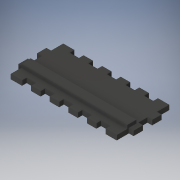
# Autodesk Inventor part: front
Saved by Autodesk Inventor 2019 (Build 230136000, 136)
## iProperties
Created: 2018-06-06
Part Number: front
Material: PBT Plastic Black
Document SubType Name: Modeling
Designer: stra92745
Density: 1.31 g/cm^3
Appearance: Smooth - White
Author: stra92745
Autodesk Inventor part; units mm, degrees
ref_plane "YZ Plane" through (0, 0, 0) normal (1, 0, 0) x (0, 1, 0)
ref_plane "XZ Plane" through (0, 0, 0) normal (0, 1, 0) x (-1, 0, 0)
ref_plane "XY Plane" through (0, 0, 0) normal (0, 0, 1) x (1, 0, 0)
sketch "Sketch1" plane through (0, 0, 0) normal (0, 1, 0) x (-1, 0, 0)
  line L0 (0, 0) -> (-99, 0)
  line L1 (-99, 0) -> (-99, -45)
  line L2 (-99, -45) -> (0, -45)
  line L3 (0, -45) -> (0, 0)
  dimension "d0" = 99
  dimension "d1" = 45
  constraints: 8 end point, 2 parallel, 1 horizontal, 1 perpendicular
  measures "d0" distance of L2.end L1.end
  measures "d1" distance of L1.end L0.end
extrude "Extrusion1" add sketch "Sketch1" along normal blind 4
sketch "Sketch2" plane through (0, 4, 0) normal (0, 1, 0) x (1, 0, 0)
  line L0 (99, 45) -> (0, 45) construction
  line L1 (99, 0) -> (99, 45) construction
  line L2 (0, 0) -> (99, 0) construction
  line L3 (0, 45) -> (0, 0) construction
  line L4 (4, 41) -> (95, 41) construction
  line L5 (95, 41) -> (95, 4) construction
  line L6 (95, 4) -> (4, 4) construction
  line L7 (4, 4) -> (4, 41) construction
  line L8 (4, 34.5) -> (0, 34.5)
  line L9 (0, 34.5) -> (0, 45)
  line L10 (0, 45) -> (4, 45)
  line L11 (4, 45) -> (4, 34.5)
  line L12 (0, 22.5) -> (99, 22.5) construction
  line L13 (49.5, 0) -> (49.5, 45) construction
  line L14 (0, 26.5) -> (4, 26.5)
  line L15 (0, 26.5) -> (0, 22.5)
  line L16 (4, 26.5) -> (4, 22.5)
  line L17 (13.5, 45) -> (13.5, 41)
  line L18 (13.5, 41) -> (21.5, 41)
  line L19 (21.5, 41) -> (21.5, 45)
  line L20 (21.5, 45) -> (13.5, 45)
  line L21 (29.5, 45) -> (29.5, 41)
  line L22 (29.5, 41) -> (37.5, 41)
  line L23 (37.5, 45) -> (37.5, 41)
  line L24 (37.5, 45) -> (29.5, 45)
  line L25 (45.5, 41) -> (45.5, 45)
  line L26 (45.5, 41) -> (49.5, 41)
  line L27 (49.5, 45) -> (45.5, 45)
  line L28 (4, 10.5) -> (0, 10.5)
  line L29 (0, 10.5) -> (0, 0)
  line L30 (0, 0) -> (4, 0)
  line L31 (4, 0) -> (4, 10.5)
  line L32 (0, 18.5) -> (4, 18.5)
  line L33 (0, 18.5) -> (0, 22.5)
  line L34 (4, 18.5) -> (4, 22.5)
  line L35 (13.5, 0) -> (13.5, 4)
  line L36 (13.5, 4) -> (21.5, 4)
  line L37 (21.5, 4) -> (21.5, 0)
  line L38 (21.5, 0) -> (13.5, 0)
  line L39 (29.5, 0) -> (29.5, 4)
  line L40 (29.5, 4) -> (37.5, 4)
  line L41 (37.5, 0) -> (37.5, 4)
  line L42 (37.5, 0) -> (29.5, 0)
  line L43 (45.5, 4) -> (45.5, 0)
  line L44 (45.5, 4) -> (49.5, 4)
  line L45 (49.5, 0) -> (45.5, 0)
  line L46 (99, 45) -> (99, 0) construction
  line L47 (95, 4) -> (95, 41) construction
  line L48 (95, 34.5) -> (99, 34.5)
  line L49 (99, 34.5) -> (99, 45)
  line L50 (99, 45) -> (95, 45)
  line L51 (95, 45) -> (95, 34.5)
  line L52 (99, 26.5) -> (95, 26.5)
  line L53 (99, 26.5) -> (99, 22.5)
  line L54 (95, 26.5) -> (95, 22.5)
  line L55 (85.5, 45) -> (85.5, 41)
  line L56 (85.5, 41) -> (77.5, 41)
  line L57 (77.5, 41) -> (77.5, 45)
  line L58 (77.5, 45) -> (85.5, 45)
  line L59 (69.5, 45) -> (69.5, 41)
  line L60 (69.5, 41) -> (61.5, 41)
  line L61 (61.5, 45) -> (61.5, 41)
  line L62 (61.5, 45) -> (69.5, 45)
  line L63 (53.5, 41) -> (53.5, 45)
  line L64 (53.5, 41) -> (49.5, 41)
  line L65 (49.5, 45) -> (53.5, 45)
  line L66 (99, 0) -> (95, 0)
  line L67 (69.5, 0) -> (69.5, 4)
  line L68 (69.5, 4) -> (61.5, 4)
  line L69 (61.5, 0) -> (69.5, 0)
  line L70 (61.5, 0) -> (61.5, 4)
  line L71 (53.5, 4) -> (53.5, 0)
  line L72 (53.5, 4) -> (49.5, 4)
  line L73 (49.5, 0) -> (53.5, 0)
  line L74 (95, 0) -> (95, 10.5)
  line L75 (95, 10.5) -> (99, 10.5)
  line L76 (99, 10.5) -> (99, 0)
  line L77 (85.5, 0) -> (85.5, 4)
  line L78 (99, 18.5) -> (95, 18.5)
  line L79 (77.5, 0) -> (85.5, 0)
  line L80 (77.5, 4) -> (77.5, 0)
  line L81 (85.5, 4) -> (77.5, 4)
  line L82 (95, 18.5) -> (95, 22.5)
  line L83 (99, 18.5) -> (99, 22.5)
  dimension "d8" = 4
  dimension "d11" = 8
  dimension "d12" = 4
  dimension "d14" = 8
  dimension "d15" = 8
  dimension "d16" = 8
  dimension "d17" = 4
  dimension "d18" = 8
  constraints: 160 end point, 49 symmetric about line, 18 point on line, 8 midpoint, 5 perpendicular, 3 collinear, 2 horizontal, 2 vertical, 1 parallel, 11 other
  measures "d11" distance between parallel lines of L14 L8
  measures "d12" distance of L14.start L15.end
  measures "d14" distance of L17.end L18.end
  measures "d15" distance between parallel lines of L21 L19
  measures "d16" distance of L21.end L22.end
  measures "d17" distance of L25.start L26.end
  measures "d18" distance between parallel lines of L23 L25
extrude "Extrusion2" cut sketch "Sketch2" against normal up to surface (4 mm away)
sketch "Sketch3" plane through (0, 4, 0) normal (0, 1, 0) x (1, 0, 0)
  line L0 (4, 10.5) -> (4, 0) projected
  line L1 (4, 9) -> (95, 9)
  line L2 (95, 9) -> (95, 17)
  line L3 (95, 17) -> (4, 17)
  line L4 (4, 17) -> (4, 9)
  line L5 (13.5, 4) -> (21.5, 4) projected
  point P0 (0, 0)
  dimension "d21" = 8
  dimension "d22" = 5
  constraints: 8 end point, 2 parallel, 1 horizontal, 1 perpendicular, 1 point on line
  measures "d21" distance of L1.end L2.end
  measures "d22" distance between parallel lines of L1 L5
extrude "Extrusion3" add sketch "Sketch3" along normal blind 3
body "Solid1"
